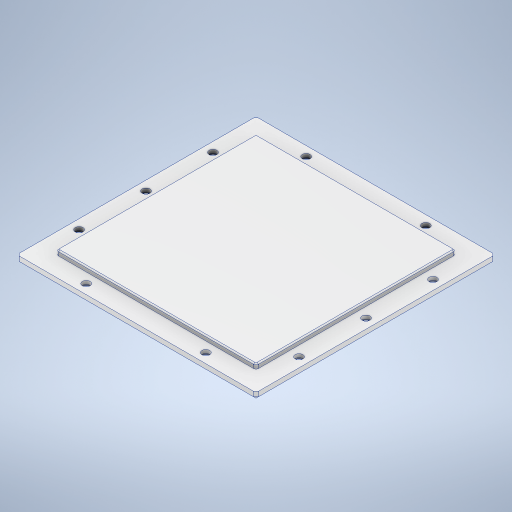
# Autodesk Inventor part: TopPanel
Saved by Autodesk Inventor 2023 (Build 270158000, 158)
## iProperties
Created: 2022-08-01
Part Number: TopPanel
Material: Aluminum 6061
Document SubType Name: Modeling
Designer: Aditya Bansal
Density: 2.7 g/cm^3
Appearance: Aluminum - Flat
Author: Aditya Bansal
Autodesk Inventor part; units mm, degrees
ref_plane "YZ Plane" through (0, 0, 0) normal (1, 0, 0) x (0, 1, 0)
ref_plane "XZ Plane" through (0, 0, 0) normal (0, 1, 0) x (-1, 0, 0)
ref_plane "XY Plane" through (0, 0, 0) normal (0, 0, 1) x (1, 0, 0)
sketch "Sketch1" plane through (0, 0, 0) normal (0, 1, 0) x (-1, 0, 0)
  line L0 (0, 0) -> (100, 0)
  line L1 (100, 0) -> (100, -100)
  line L2 (100, -100) -> (0, -100)
  line L3 (0, -100) -> (0, 0)
  dimension "d0" = 100
  constraints: 8 end point, 2 parallel, 2 perpendicular, 1 horizontal
  measures "d0" distance of L0.end L1.end
extrude "Extrusion1" add sketch "Sketch1" along normal blind 3
sketch "Sketch2" plane through (0, 3, 0) normal (0, 1, 0) x (1, 0, 0)
  line L0 (-100, 100) -> (0, 100) construction
  line L1 (0, 100) -> (0, 92) construction
  line L2 (0, 92) -> (-100, 92) construction
  line L3 (-100, 92) -> (-100, 100) construction
  line L4 (-100, 0) -> (0, 0) construction
  line L5 (0, 0) -> (0, 8) construction
  line L6 (0, 8) -> (-100, 8) construction
  line L7 (-100, 8) -> (-100, 0) construction
  line L8 (-100, 92) -> (-92, 92) construction
  line L9 (-92, 92) -> (-92, 8) construction
  line L10 (-92, 8) -> (-100, 8) construction
  line L11 (-100, 8) -> (-100, 92) construction
  line L12 (0, 8) -> (-8, 8) construction
  line L13 (-8, 8) -> (-8, 92) construction
  line L14 (-8, 92) -> (0, 92) construction
  line L15 (0, 92) -> (0, 8) construction
  line L16 (-91.75, 91.75) -> (-8.25, 91.75)
  line L17 (-8.25, 91.75) -> (-8.25, 8.25)
  line L18 (-8.25, 8.25) -> (-91.75, 8.25)
  line L19 (-91.75, 8.25) -> (-91.75, 91.75)
  point P0 (0, 0)
  dimension "d24" = 8
  dimension "d25" = 8
  dimension "d26" = 0.25
  dimension "d27" = 0.25
  dimension "d28" = 0.25
  dimension "d29" = 0.25
  constraints: 40 end point, 10 parallel, 5 horizontal, 5 perpendicular, 3 collinear, 2 point on line, 1 coincident
  measures "d24" distance between parallel lines of L15 L13
  measures "d25" distance between parallel lines of L0 L2
  measures "d26" distance between parallel lines of L9 L19
  measures "d27" distance between parallel lines of L2 L16
  measures "d28" distance between parallel lines of L13 L17
  measures "d29" distance between parallel lines of L6 L18
extrude "Extrusion2" add sketch "Sketch2" along normal blind 2
sketch "Sketch4" plane through (0, 0, 0) normal (0, -1, 0) x (1, 0, 0)
  line L0 (-91.75, -8.25) -> (-8.25, -8.25) projected
  line L1 (-8.25, -8.25) -> (-8.25, -91.75) projected
  line L2 (-8.25, -91.75) -> (-91.75, -91.75) projected
  line L3 (-91.75, -91.75) -> (-91.75, -8.25) projected
  line L4 (0, -100) -> (-100, -100) projected
  line L5 (0, 0) -> (0, -100) projected
  line L6 (-100, 0) -> (0, 0) projected
  line L7 (-100, -100) -> (-100, 0) projected
  point P0 (-4, -78)
  point P1 (-4, -22)
  point P2 (-96, -22)
  point P3 (-96, -78)
  point P4 (-96, -50)
  point P5 (-4, -50)
  point P6 (-25, -96)
  point P7 (-75, -96)
  point P8 (-75, -4)
  point P9 (-25, -4)
  dimension "d49" = 8.25
  dimension "d50" = 4
  dimension "d51" = 4
  dimension "d52" = 83.5
  dimension "d57" = 8.25
  dimension "d58" = 4
  dimension "d59" = 4
  dimension "d60" = 100
  dimension "d61" = 25
  dimension "d62" = 50
  dimension "d63" = 13.75
  dimension "d64" = 28
  dimension "d65" = 28
  dimension "d66" = 13.75
  constraints: 6 vertical alignment, 5 horizontal alignment
  measures "d49" distance between parallel lines of L1 L5
  measures "d50" distance from line of point (-4, -78) L5
  measures "d51" distance from line of L7 point (-96, -78)
  measures "d52" distance of L0.end L1.end
  measures "d57" distance between parallel lines of L4 L2
  measures "d58" distance from line of L4 point (-75, -96)
  measures "d59" distance from line of L6 point (-75, -4)
  measures "d60" distance of L6.start L5.start
  measures "d61" distance from line of point (-25, -4) L5
  measures "d62" distance of point (-75, -4) point (-25, -4)
  measures "d63" distance from line of point (-4, -78) L2
  measures "d64" distance of point (-4, -50) point (-4, -78)
  measures "d65" distance of point (-4, -22) point (-4, -50)
  measures "d66" distance from line of L0 point (-4, -22)
hole "Hole2" at (-4, 0, -78) at (-4, 0, -50) at (-4, 0, -22) at (-96, 0, -22) at (-96, 0, -50) at (-96, 0, -78) at (-25, 0, -4) at (-75, 0, -4) at (-25, 0, -96) at (-75, 0, -96) direction (0, 1, 0) diameter 3.2 depth 3 countersink diameter 6.3 countersink angle 90 clearance for "Flat Head Machine Screw" size "M3" standard "Ansi Metric M Profile"
fillet "Fillet3" radius 1 4 edges at (-91.75, 4, -91.75) (-8.25, 4, -91.75) (-91.75, 4, -8.25) (-8.25, 4, -8.25)
chamfer "Chamfer2" distance 0.5 angle 45 4 edges at (-91.75, 5, -50) (-50, 5, -8.25) (-8.25, 5, -50) (-50, 5, -91.75)
chamfer "Chamfer3" distance 1 angle 45 8 edges at (-50, 0, 0) (0, 0, -50) (-100, 0, -50) (-50, 0, -100) (0, 1.5, -100) (0, 1.5, 0) (-100, 1.5, 0) (-100, 1.5, -100)
equation "\"d27\" = d26"
equation "\"d28\" = d26"
equation "\"d29\" = d28"
body "Solid1"
